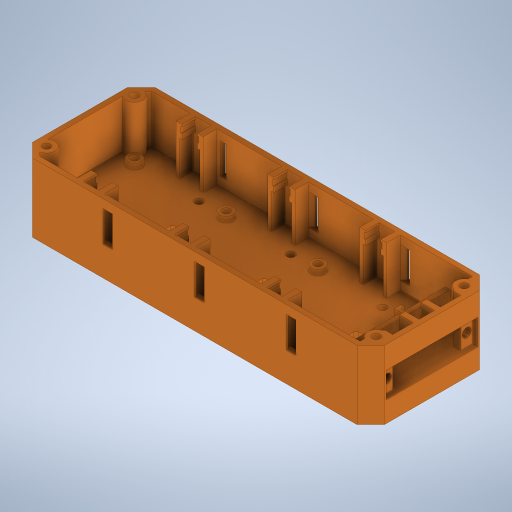
# Autodesk Inventor part: Sujecion
Saved by Autodesk Inventor 2024.2 (Build 282272000, 272)
## iProperties
Created: 2024-08-10
Part Number: Sujecion
Material: Generic
Document SubType Name: Modeling
Designer: Admin
Density: 1 g/cm^3
Appearance: Metal 1600F Hot
Author: Admin
Autodesk Inventor part; units mm, degrees
ref_plane "YZ Plane" through (0, 0, 0) normal (1, 0, 0) x (0, 1, 0)
ref_plane "XZ Plane" through (0, 0, 0) normal (0, 1, 0) x (-1, 0, 0)
sketch "Sketch1" plane through (0, 0, 0) normal (0, 1, 0) x (-1, 0, 0)
  line L0 (0, 0) -> (64, 0)
  line L1 (64, 0) -> (64, -72)
  line L2 (64, -72) -> (0, -72)
  line L3 (0, -72) -> (0, 0) construction
  line L4 (0, 0) -> (64, -72) construction
  line L5 (51, -17) -> (13, -17)
  line L6 (13, -17) -> (13, -55)
  line L7 (13, -55) -> (51, -55)
  line L8 (51, -55) -> (51, -17)
  line L9 (51, -17) -> (13, -55) construction
  line L10 (13, -17) -> (51, -55) construction
  circle A0 centre (51, -55) radius 1.6
  circle A1 centre (51, -17) radius 1.6
  circle A2 centre (13, -17) radius 1.6
  line L11 (10, -58) -> (54, -58) construction
  line L12 (54, -58) -> (54, -14) construction
  line L13 (54, -14) -> (10, -14) construction
  line L14 (10, -14) -> (10, -58) construction
  line L15 (10, -58) -> (54, -14) construction
  line L16 (54, -58) -> (10, -14) construction
  circle A3 centre (13, -55) radius 2.275
  circle A4 centre (-41, -55) radius 2.275
  line L17 (-41, -55) -> (-3, -55)
  circle A5 centre (-3, -55) radius 1.6
  line L18 (-44, -58) -> (0, -58) construction
  line L19 (-41, -17) -> (-41, -55)
  circle A6 centre (-41, -17) radius 1.6
  line L20 (-44, -14) -> (-44, -58) construction
  line L21 (10, -72) -> (-54, -72)
  line L22 (-3, -17) -> (-41, -55) construction
  line L23 (-3, -17) -> (-41, -17)
  line L24 (-3, -55) -> (-3, -17)
  line L25 (0, -58) -> (0, -14) construction
  line L26 (-44, -58) -> (0, -14) construction
  line L27 (0, -58) -> (-44, -14) construction
  line L28 (-54, -72) -> (-54, 0) construction
  line L29 (-54, 0) -> (10, -72) construction
  line L30 (-54, 0) -> (10, 0)
  line L31 (-41, -17) -> (-3, -55) construction
  circle A7 centre (-3, -17) radius 1.6
  line L32 (0, -14) -> (-44, -14) construction
  circle A8 centre (-95, -55) radius 2.275
  line L33 (-95, -55) -> (-57, -55)
  circle A9 centre (-57, -55) radius 1.6
  line L34 (-98, -58) -> (-54, -58) construction
  line L35 (-95, -17) -> (-95, -55)
  circle A10 centre (-95, -17) radius 1.6
  line L36 (-98, -14) -> (-98, -58) construction
  line L37 (-44, -72) -> (-108, -72)
  line L38 (-57, -17) -> (-95, -55) construction
  line L39 (-57, -17) -> (-95, -17)
  line L40 (-57, -55) -> (-57, -17)
  line L41 (-54, -58) -> (-54, -14) construction
  line L42 (-98, -58) -> (-54, -14) construction
  line L43 (-54, -58) -> (-98, -14) construction
  line L44 (-108, -72) -> (-108, 0) construction
  line L45 (-108, 0) -> (-44, -72) construction
  line L46 (-108, 0) -> (-44, 0)
  line L47 (-95, -17) -> (-57, -55) construction
  circle A11 centre (-57, -17) radius 1.6
  line L48 (-54, -14) -> (-98, -14) construction
  line L49 (-108, 0) -> (-143, 0)
  line L50 (-143, 0) -> (-143, -72)
  line L51 (-143, -72) -> (-108, -72)
  line L52 (-108, -72) -> (-108, 0) construction
  point P0 (32, -36)
  point P1 (-22, -36)
  point P2 (-76, -36)
  dimension "d0" = 64
  dimension "d1" = 72
  dimension "d2" = 38
  dimension "d3" = 38
  dimension "d6" = 3.2
  dimension "d9" = 180
  dimension "d11" = 44
  dimension "d12" = 44
  dimension "d13" = 4.55
  dimension "d21" = 54
  dimension "d26" = 35
  constraints: 106 end point, 12 centre point, 8 parallel, 6 coincident, 5 horizontal, 5 midpoint, 4 perpendicular, 1 collinear, 78 other
  measures "d0" distance of L0.start L0.end
  measures "d1" distance of L0.end L1.end
  measures "d2" distance of L7.end L5.start
  measures "d3" distance of L6.end L7.end
  measures "d6" diameter of A0
  measures "d11" distance of L13.end L12.end
  measures "d12" distance of L12.end L11.end
  measures "d13" diameter of A3
  measures "d21" distance of A3.centre A4.centre
  measures "d26" distance of L51.end L50.end
extrude "Base" add sketch "Sketch1" along normal blind 3.2 contours L0 L1 L2 L21 L37 L51 L50 L49 L46 L30 | L5 A1 L8 A0 L7 A3 L6 A2 | A4 L19 A6 L23 A7 L24 A5 L17 | A8 L35 A10 L39 A11 L40 A9 L33
sketch "Sketch2" plane through (0, 3.2, 0) normal (0, 1, 0) x (1, 0, 0)
  circle A0 centre (-13, 17) radius 1.6 projected
  line L0 (-13, 17) -> (-51, 55) construction
  circle A1 centre (-51, 55) radius 2.25
  circle A2 centre (-51, 55) radius 4
  line L1 (-32, 36) -> (-39.676, 28.324) construction
  circle A3 centre (-51, 17) radius 4
  circle A4 centre (-51, 17) radius 2.25
  circle A5 centre (-13, 17) radius 4
  circle A6 centre (-13, 17) radius 2.25
  line L2 (-64, 0) -> (143, 0) projected
  line L3 (-64, 0) -> (-54, 0)
  circle A7 centre (3, 17) radius 4
  circle A8 centre (3, 17) radius 2.25
  circle A9 centre (41, 17) radius 4
  circle A10 centre (41, 17) radius 2.25
  circle A11 centre (3, 55) radius 4
  circle A12 centre (3, 55) radius 2.25
  circle A13 centre (57, 17) radius 4
  circle A14 centre (57, 17) radius 2.25
  circle A15 centre (95, 17) radius 4
  circle A16 centre (95, 17) radius 2.25
  circle A17 centre (57, 55) radius 4
  circle A18 centre (57, 55) radius 2.25
  point P0 (0, 0)
  dimension "d29" = 4.5
  dimension "d30" = 8
  dimension "d33" = 180
  dimension "d38" = 54
  constraints: 18 centre point, 10 coincident, 6 end point, 1 horizontal, 1 midpoint, 1 point on line, 33 other
  measures "d29" diameter of A1
  measures "d30" diameter of A2
  measures "d38" distance of A3.centre A7.centre
extrude "EspacioInsertos" add sketch "Sketch2" along normal blind 3.2 contours A2 | A3 | A5 | A7 | A9 | A11 | A13 | A15 | A17
sketch "Sketch3" plane through (0, 3.2, 0) normal (0, 1, 0) x (1, 0, 0)
  circle A0 centre (-13, 17) radius 2.25 construction
  circle A1 centre (-51, 55) radius 2.25 construction
  line L0 (-13, 17) -> (-51, 55) construction
  line L1 (-54, 14) -> (-10, 14) construction
  line L2 (-10, 14) -> (-10, 58) construction
  line L3 (-10, 58) -> (-54, 58) construction
  line L4 (-54, 58) -> (-54, 14) construction
  line L5 (-54, 14) -> (-10, 58) construction
  line L6 (-10, 14) -> (-54, 58) construction
  line L7 (-9, 20.1) -> (-2.5, 20.1)
  line L8 (-2.5, 20.1) -> (-2.5, 35.6)
  line L9 (-2.5, 35.6) -> (-9, 35.6)
  line L10 (-9, 35.6) -> (-9, 20.1)
  line L11 (-9, 20.1) -> (-2.5, 35.6) construction
  line L12 (-2.5, 20.1) -> (-9, 35.6) construction
  line L13 (-64, 0) -> (143, 0) projected
  line L14 (-9, 21.6) -> (-7.5, 20.1)
  line L15 (-5.75, 27.85) -> (-7.0439, 27.85) construction
  line L16 (-5.75, 27.85) -> (-5.75, 26.4341) construction
  line L17 (-9, 34.1) -> (-7.5, 35.6)
  line L18 (-2.5, 21.6) -> (-4, 20.1)
  line L19 (-2.5, 34.1) -> (-4, 35.6)
  line L20 (45, 21.6) -> (46.5, 20.1)
  line L21 (45, 35.6) -> (45, 20.1)
  line L22 (45, 20.1) -> (51.5, 20.1)
  line L23 (51.5, 21.6) -> (50, 20.1)
  line L24 (51.5, 20.1) -> (51.5, 35.6)
  line L25 (51.5, 34.1) -> (50, 35.6)
  line L26 (51.5, 35.6) -> (45, 35.6)
  line L27 (45, 34.1) -> (46.5, 35.6)
  line L28 (0, 58) -> (0, 14) construction
  line L29 (0, 14) -> (44, 14) construction
  line L30 (44, 58) -> (0, 58) construction
  line L31 (44, 14) -> (44, 58) construction
  line L32 (99, 21.6) -> (100.5, 20.1)
  line L33 (99, 35.6) -> (99, 20.1)
  line L34 (99, 20.1) -> (105.5, 20.1)
  line L35 (105.5, 21.6) -> (104, 20.1)
  line L36 (105.5, 20.1) -> (105.5, 35.6)
  line L37 (105.5, 34.1) -> (104, 35.6)
  line L38 (105.5, 35.6) -> (99, 35.6)
  line L39 (99, 34.1) -> (100.5, 35.6)
  line L40 (54, 58) -> (54, 14) construction
  line L41 (54, 14) -> (98, 14) construction
  line L42 (98, 58) -> (54, 58) construction
  line L43 (98, 14) -> (98, 58) construction
  point P0 (0, 0)
  point P1 (-32, 36)
  dimension "d45" = 44
  dimension "d46" = 44
  dimension "d47" = 15.5
  dimension "d48" = 6.5
  dimension "d49" = 20.1
  dimension "d50" = 1
  dimension "d51" = 135
  dimension "d52" = 1.5
  dimension "d55" = 54
  constraints: 86 end point, 6 point on line, 6 symmetric about line, 5 midpoint, 4 parallel, 3 horizontal, 3 perpendicular, 1 vertical, 56 other
  measures "d45" distance of L3.end L2.end
  measures "d46" distance of L2.end L1.end
  measures "d47" distance of L9.end L7.start
  measures "d48" distance of L8.end L9.end
  measures "d49" distance between parallel lines of L13 L7
  measures "d50" distance between parallel lines of L10 L2
  measures "d51" angle of L14 L10
  measures "d52" horizontal distance of L14.start L14.end
  measures "d55" distance of L14.start L20.start
extrude "EntradaCables" cut sketch "Sketch3" against normal blind 3.2 contours L14 L10 L17 L9 L19 L8 L18 L7 | L21 L27 L26 L25 L24 L23 L22 L20 | L33 L39 L38 L37 L36 L35 L34 L32
sketch "Sketch4" plane through (0, 3.2, 0) normal (0, 1, 0) x (1, 0, 0)
  line L0 (-64, 72) -> (-64, 0) projected
  line L1 (143, 0) -> (143, 72) projected
  line L2 (-64, 72) -> (143, 72)
  line L3 (143, 72) -> (143, 0)
  line L4 (143, 0) -> (-64, 0)
  line L5 (-64, 0) -> (-64, 72)
  line L6 (143, 72) -> (-64, 72) projected
  line L7 (39.5, 72) -> (39.5, 36) construction
  line L8 (140, 69) -> (-61, 69)
  line L9 (-61, 69) -> (-61, 3)
  line L10 (-61, 3) -> (140, 3)
  line L11 (140, 3) -> (140, 69)
  line L12 (140, 69) -> (-61, 3) construction
  line L13 (-61, 69) -> (140, 3) construction
  point P0 (0, 0)
  dimension "d62" = 3
  dimension "d63" = 3
  dimension "d64" = 3
  constraints: 22 end point, 4 parallel, 3 midpoint, 2 horizontal, 2 perpendicular, 1 vertical
  measures "d62" distance between parallel lines of L9 L0
  measures "d63" distance between parallel lines of L4 L10
  measures "d64" distance between parallel lines of L2 L8
extrude "EliminacionExceso" add sketch "Sketch4" along normal blind 30
sketch "Sketch5" plane through (0, 3.2, 0) normal (0, 1, 0) x (1, 0, 0)
  circle A0 centre (-13, 17) radius 1.6 projected
  circle A1 centre (-51, 55) radius 4 projected
  line L0 (-13, 17) -> (-51, 55) construction
  line L1 (-54, 14) -> (-10, 14)
  line L2 (-10, 14) -> (-10, 58)
  line L3 (-10, 58) -> (-54, 58)
  line L4 (-54, 58) -> (-54, 14)
  line L5 (-54, 14) -> (-10, 58) construction
  line L6 (-10, 14) -> (-54, 58) construction
  line L7 (-61, 3) -> (140, 3) projected
  line L8 (-32.5, 3) -> (-16.5, 3)
  line L9 (-16.5, 3) -> (-16.5, 11)
  line L10 (-16.5, 11) -> (-32.5, 11)
  line L11 (-32.5, 11) -> (-32.5, 3)
  line L12 (37.5, 3) -> (37.5, 11)
  line L13 (37.5, 11) -> (21.5, 11)
  line L14 (21.5, 11) -> (21.5, 3)
  line L15 (21.5, 3) -> (37.5, 3)
  line L16 (91.5, 3) -> (91.5, 11)
  line L17 (91.5, 11) -> (75.5, 11)
  line L18 (75.5, 11) -> (75.5, 3)
  line L19 (75.5, 3) -> (91.5, 3)
  line L20 (143, 0) -> (143, 72) projected
  line L21 (143, 36) -> (123, 36) construction
  line L22 (-61, 69) -> (140, 69)
  line L23 (-32.5, 69) -> (-16.5, 69)
  line L24 (-16.5, 69) -> (-16.5, 61)
  line L25 (-16.5, 61) -> (-32.5, 61)
  line L26 (-32.5, 61) -> (-32.5, 69)
  line L27 (37.5, 69) -> (37.5, 61)
  line L28 (37.5, 61) -> (21.5, 61)
  line L29 (21.5, 61) -> (21.5, 69)
  line L30 (21.5, 69) -> (37.5, 69)
  line L31 (91.5, 69) -> (91.5, 61)
  line L32 (91.5, 61) -> (75.5, 61)
  line L33 (75.5, 61) -> (75.5, 69)
  line L34 (75.5, 69) -> (91.5, 69)
  point P0 (0, 0)
  point P1 (-32, 36)
  point P2 (91.5, 69)
  point P3 (75.5, 69)
  point P4 (37.5, 69)
  point P5 (21.5, 69)
  point P6 (-16.5, 69)
  dimension "d67" = 44
  dimension "d68" = 44
  dimension "d69" = 21.5
  dimension "d70" = 8
  dimension "d71" = 16
  dimension "d74" = 54
  constraints: 66 end point, 14 symmetric about line, 4 horizontal, 4 midpoint, 4 parallel, 2 perpendicular, 2 point on line, 16 other
  measures "d67" distance of L3.end L2.end
  measures "d68" distance of L2.end L1.end
  measures "d69" distance between parallel lines of L11 L4
  measures "d70" distance of L10.end L8.start
  measures "d71" distance of L9.end L10.end
  measures "d74" distance of L8.start L14.end
extrude "EspacioConectores" add sketch "Sketch5" along normal blind 30 contours L11 L10 L9 L7 | L14 L13 L12 L7 | L18 L17 L16 L7 | L22 L24 L25 L26 | L22 L27 L28 L29 | L22 L31 L32 L33
sketch "Sketch6" plane through (-16.5, 3.2, -11) normal (0, 0, -1) x (-1, 0, 0)
  line L0 (16, 0) -> (16, 30) projected
  line L1 (0, 0) -> (0, 30) projected
  line L2 (8, 30) -> (8, 27)
  line L3 (8, 30) -> (12.5, 30)
  line L4 (12.5, 30) -> (12.5, 27)
  line L5 (12.5, 27) -> (8, 27)
  line L6 (8, 27) -> (8, 30)
  line L7 (8, 27) -> (13.2, 27)
  line L8 (13.2, 27) -> (13.2, 23.5)
  line L9 (13.2, 23.5) -> (8, 23.5)
  line L10 (8, 23.5) -> (8, 27)
  line L11 (8, 23.5) -> (12.5, 23.5)
  line L12 (12.5, 23.5) -> (12.5, 20.5)
  line L13 (12.5, 20.5) -> (8, 20.5)
  line L14 (8, 20.5) -> (8, 23.5)
  line L15 (16, 0) -> (0, 0) projected
  line L16 (8, 20.5) -> (14, 20.5)
  line L17 (14, 20.5) -> (14, 0)
  line L18 (14, 0) -> (8, 0)
  line L19 (8, 0) -> (8, 20.5)
  line L20 (0, 0) -> (0, 30)
  line L21 (8, 30) -> (3.5, 30)
  line L22 (3.5, 30) -> (3.5, 27)
  line L23 (3.5, 27) -> (8, 27)
  line L24 (8, 27) -> (2.8, 27)
  line L25 (2.8, 27) -> (2.8, 23.5)
  line L26 (2.8, 23.5) -> (8, 23.5)
  line L27 (8, 23.5) -> (3.5, 23.5)
  line L28 (3.5, 23.5) -> (3.5, 20.5)
  line L29 (3.5, 20.5) -> (8, 20.5)
  line L30 (0, 0) -> (16, 0)
  line L31 (8, 20.5) -> (2, 20.5)
  line L32 (2, 20.5) -> (2, 0)
  line L33 (2, 0) -> (8, 0)
  point P0 (-16.5, -3.2)
  point P1 (2, 0)
  point P2 (12.5, 23.5)
  point P3 (3.5, 23.5)
  dimension "d84" = 4.5
  dimension "d85" = 5.2
  dimension "d86" = 3.5
  dimension "d88" = 3
  dimension "d89" = 3
  dimension "d90" = 6
  constraints: 62 end point, 10 symmetric about line, 8 parallel, 4 horizontal, 4 perpendicular, 2 point on line, 1 vertical
  measures "d84" distance of L4.end L5.end
  measures "d85" distance of L8.end L9.end
  measures "d86" distance of L7.end L8.end
  measures "d88" distance between parallel lines of L7 L3
  measures "d89" distance of L11.end L12.end
  measures "d90" distance of L17.end L18.end
extrude "EntradaConectores" cut sketch "Sketch6" against normal blind 8
pattern_linear "PatronConectoresI" count 3 spacing 54 along (1, 0, 0) of "EntradaConectores"
ref_plane "PlanoDivisor" through (0, 0, -36) normal (0, 0, 1) x (1, 0, 0)
mirror "PatronConectoresII" about plane through (0, 0, -36) normal (0, 0, 1) of "EntradaConectores", "PatronConectoresI"
sketch "Sketch7" plane through (0, 33.2, 0) normal (0, 1, 0) x (1, 0, 0)
  line L0 (-64, 0) -> (143, 0) projected
  line L1 (143, 0) -> (-64, 0)
  line L2 (-64, 0) -> (-64, 72)
  line L3 (-64, 72) -> (143, 72)
  line L4 (143, 72) -> (143, 0)
  point P0 (0, 0)
  constraints: 8 end point, 2 parallel, 1 horizontal, 1 perpendicular
extrude "DetalleSuperficialI" cut sketch "Sketch7" against normal blind 1.8
sketch "Sketch8" plane through (0, 3.2, 0) normal (0, 1, 0) x (1, 0, 0)
  line L0 (-64, 0) -> (-64, 72) projected
  line L1 (-64, 8) -> (-56, 0)
  line L2 (143, 0) -> (-64, 0) projected
  line L3 (-64, 8) -> (-64, 0)
  line L4 (-56, 0) -> (-64, 0)
  line L5 (-64, 36) -> (-49, 36) construction
  line L6 (-64, 12.2426) -> (-51.7574, 0)
  line L7 (-64, 72) -> (-64, 0)
  line L8 (-64, 64) -> (-56, 72)
  line L9 (143, 72) -> (-64, 72)
  line L10 (-64, 64) -> (-64, 72)
  line L11 (-56, 72) -> (-64, 72)
  line L12 (-64, 59.7574) -> (-51.7574, 72)
  line L13 (39.5, 72) -> (39.5, 42) construction
  line L14 (143, 0) -> (143, 72)
  line L15 (143, 8) -> (135, 0)
  line L16 (-64, 0) -> (143, 0)
  line L17 (143, 8) -> (143, 0)
  line L18 (135, 0) -> (143, 0)
  line L19 (143, 36) -> (128, 36) construction
  line L20 (143, 12.2426) -> (130.7574, 0)
  line L21 (143, 72) -> (143, 0)
  line L22 (143, 64) -> (135, 72)
  line L23 (-64, 72) -> (143, 72)
  line L24 (143, 64) -> (143, 72)
  line L25 (135, 72) -> (143, 72)
  line L26 (143, 59.7574) -> (130.7574, 72)
  point P0 (0, 0)
  point P1 (130.7574, 0)
  dimension "d99" = 135
  dimension "d100" = 8
  dimension "d102" = 3
  constraints: 50 end point, 23 symmetric about line, 16 point on line, 2 collinear, 2 midpoint, 1 horizontal, 1 parallel, 1 vertical
  measures "d99" angle of L0 L1
  measures "d100" horizontal distance of L1.start L1.end
  measures "d102" distance between parallel lines of L6 L1
extrude "DetalleSuperficialII" cut sketch "Sketch8" along normal through all both and the other way through all contours L0 L1 L2 | L0 L9 L8 | L15 L14 L2 | L9 L14 L22
extrude "Extrusion9" add sketch "Sketch8" along normal blind 28.2 contours L0 L6 L2 L1 | L0 L8 L9 L12 | L20 L14 L15 L2 | L9 L22 L14 L26
sketch "Sketch14" plane through (0, 3.2, 0) normal (0, 1, 0) x (1, 0, 0)
  line L0 (135, 72) -> (-56, 72) projected
  line L1 (121, 72) -> (121, 0)
  line L2 (143, 64) -> (143, 8) projected
  line L3 (118, 72) -> (118, 0)
  line L4 (118, 72) -> (121, 72)
  line L5 (118, 0) -> (121, 0)
  point P0 (0, 0)
  dimension "d117" = 22
  dimension "d118" = 3
  constraints: 8 end point, 2 parallel, 1 horizontal, 1 point on line, 1 vertical
  measures "d117" distance between parallel lines of L2 L1
  measures "d118" distance between parallel lines of L1 L3
extrude "EspacioFusible" add sketch "Sketch14" along normal blind 15
sketch "Sketch21" plane through (143, 0, -8) normal (1, 0, 0) x (0, 0, -1)
  line L0 (0, 31.4) -> (56, 31.4) projected
  line L1 (28, 31.4) -> (28, 0) construction
  line L2 (56, 0) -> (0, 0) projected
  line L3 (28, 0) -> (28, 3.2)
  line L4 (28, 3.2) -> (8, 3.2)
  line L5 (8, 3.2) -> (8, 18.2)
  line L6 (8, 18.2) -> (28, 18.2)
  line L7 (28, 18.2) -> (28, 3.2)
  line L8 (28, 3.2) -> (48, 3.2)
  line L9 (48, 3.2) -> (48, 18.2)
  line L10 (48, 18.2) -> (28, 18.2)
  point P0 (-8, 0)
  dimension "d138" = 3.2
  dimension "d139" = 20
  dimension "d140" = 15
  constraints: 18 end point, 2 midpoint, 2 parallel, 2 symmetric about line, 1 horizontal, 1 perpendicular, 1 point on line
  measures "d138" distance of L1.end L3.end
  measures "d139" distance of L5.end L6.end
  measures "d140" distance of L4.end L5.end
extrude "AccesoFusible" cut sketch "Sketch21" against normal blind 3
sketch "Sketch23" plane through (143, 0, -8) normal (1, 0, 0) x (0, 0, -1)
  line L0 (8, 18.2) -> (8, 3.2) construction
  line L1 (48, 3.2) -> (48, 18.2) construction
  line L2 (8, 18.2) -> (48, 18.2) construction
  line L3 (48, 18.2) -> (48, 3.2) construction
  line L4 (48, 3.2) -> (8, 3.2) construction
  line L5 (8, 3.2) -> (8, 18.2) construction
  line L6 (48, 18.2) -> (8, 3.2) construction
  circle A0 centre (28, 10.7) radius 2.25
  point P0 (-8, 0)
  dimension "d143" = 4.5
  constraints: 10 end point, 2 parallel, 1 centre point, 1 horizontal, 1 midpoint, 1 perpendicular
  measures "d143" diameter of A0
extrude "BarrenoFusible" cut sketch "Sketch23" against normal blind 30
sketch "Sketch24" plane through (0, 31.4, 0) normal (0, 1, 0) x (1, 0, 0)
  line L0 (121, 3) -> (121, 69) projected
  line L1 (121, 36) -> (131, 36) construction
  line L2 (121, 3) -> (133.7574, 3) projected
  line L3 (140, 9.2426) -> (140, 16) projected
  line L4 (133.7574, 3) -> (140, 9.2426)
  line L5 (140, 9.2426) -> (140, 16)
  line L6 (140, 16) -> (133.7574, 16)
  line L7 (133.7574, 16) -> (133.7574, 3)
  line L8 (140, 62.7574) -> (140, 56)
  line L9 (133.7574, 69) -> (140, 62.7574)
  line L10 (140, 62.7574) -> (140, 56)
  line L11 (140, 56) -> (133.7574, 56)
  line L12 (133.7574, 56) -> (133.7574, 69)
  point P0 (0, 0)
  constraints: 20 end point, 4 symmetric about line, 2 perpendicular, 1 collinear, 1 horizontal, 1 midpoint
extrude "SeccionMagnetos" add sketch "Sketch24" against normal blind 28.2
sketch "Sketch25" plane through (143, 0, -8) normal (1, 0, 0) x (0, 0, -1)
  line L0 (61, 18.2) -> (-5, 18.2) projected
  line L1 (55, 3.2) -> (1, 3.2)
  line L2 (1, 3.2) -> (1, 18.2)
  line L3 (1, 18.2) -> (55, 18.2)
  line L4 (55, 18.2) -> (55, 3.2)
  circle A0 centre (28, 10.7) radius 2.25 projected
  line L5 (55, 3.2) -> (1, 18.2) construction
  line L6 (1, 3.2) -> (55, 18.2) construction
  point P0 (-8, 0)
  dimension "d149" = 54
  constraints: 12 end point, 2 midpoint, 2 parallel, 1 horizontal, 1 perpendicular, 1 point on line
  measures "d149" distance of L2.end L3.end
extrude "EspacioTapa" cut sketch "Sketch25" against normal blind 3
sketch "Sketch28" plane through (0, 31.4, 0) normal (0, 1, 0) x (1, 0, 0)
  line L0 (-64, 64) -> (-64, 8) projected
  line L1 (-64, 36) -> (-69, 36) construction
  line L2 (-61, 9.2426) -> (-54.7574, 3) projected
  line L3 (-57.8787, 6.1213) -> (-57.8787, 65.8787) construction
  circle A0 centre (-57.8787, 10.1213) radius 2.25
  line L4 (-54.7574, 3) -> (-61, 9.2426) projected
  circle A1 centre (-57.8787, 10.1213) radius 5
  circle A2 centre (-57.8787, 61.8787) radius 2.25
  circle A3 centre (-57.8787, 61.8787) radius 5
  line L5 (0, 0) -> (-25.1943, 0) construction
  line L6 (-56, 0) -> (135, 0) projected
  circle A4 centre (136.1213, 10.1213) radius 5
  circle A5 centre (136.1213, 10.1213) radius 2.25
  circle A6 centre (136.1213, 61.8787) radius 5
  circle A7 centre (136.1213, 61.8787) radius 2.25
  dimension "d159" = 4.5
  dimension "d160" = 4
  dimension "d161" = 10
  dimension "d164" = 194
  constraints: 8 centre point, 6 end point, 3 midpoint, 2 horizontal, 2 point on line, 1 symmetric about line, 1 vertical, 8 other
  measures "d159" diameter of A0
  measures "d160" distance of point (-57.879, 6.121) A0.centre
  measures "d161" diameter of A1
  measures "d164" distance of A0.centre A4.centre
extrude "BarrenosTapaI" add sketch "Sketch28" against normal blind 28.2 contours A1 | A3
extrude "BarrenosTapaII" add sketch "Sketch28" against normal blind 10 contours A4 | A6
extrude "Extrusion25" cut sketch "Sketch28" against normal blind 10 contours A5 | A7
sketch "Sketch31" plane through (0, 0, 0) normal (0, -1, 0) x (1, 0, 0)
  line L0 (-56, 0) -> (-64, -8) projected
  line L1 (-56, 0) -> (-64, -8)
  line L2 (-64, -64) -> (-64, -8) projected
  line L3 (-64, -8) -> (-64, -64)
  line L4 (135, -72) -> (-56, -72) projected
  line L5 (-64, -64) -> (-56, -72)
  line L6 (135, -72) -> (143, -64) projected
  line L7 (-56, -72) -> (135, -72)
  line L8 (135, -72) -> (143, -64)
  line L9 (143, -64) -> (143, -8)
  line L10 (143, -8) -> (135, 0)
  line L11 (135, 0) -> (-56, 0)
  line L12 (-54.7574, -3) -> (-61, -9.2426)
  line L13 (-61, -9.2426) -> (-61, -62.7574)
  line L14 (-61, -62.7574) -> (-54.7574, -69)
  line L15 (-54.7574, -69) -> (133.7574, -69)
  line L16 (133.7574, -69) -> (140, -62.7574)
  line L17 (140, -62.7574) -> (140, -9.2426)
  line L18 (140, -9.2426) -> (133.7574, -3)
  line L19 (133.7574, -3) -> (-54.7574, -3)
  point P0 (0, 0)
  dimension "d181" = 3
  constraints: 32 end point, 8 perpendicular, 5 equal length, 7 other
  measures "d181" distance between parallel lines of L11 L19
extrude "Extrusion27" add sketch "Sketch31" along normal blind 9
sketch "Sketch26" plane through (140, 0, -8) normal (1, 0, 0) x (0, 0, -1)
  line L0 (55, 18.2) -> (55, 3.2) projected
  line L1 (1, 3.2) -> (1, 18.2) projected
  line L2 (48, 18.2) -> (8, 18.2) projected
  line L3 (8, 18.2) -> (8, 3.2) projected
  line L4 (8, 18.2) -> (8, 3.2)
  line L5 (48, 18.2) -> (48, 3.2)
  line L6 (44.725, 3.2) -> (49.275, 3.2) projected
  line L7 (55, 10.7) -> (48, 10.7) construction
  line L8 (8, 10.7) -> (1, 10.7) construction
  circle A0 centre (4.5, 10.7) radius 2.6
  line L9 (28, 18.2) -> (28, 15.2) construction
  circle A1 centre (51.5, 10.7) radius 2.6
  point P0 (-8, 0)
  dimension "d152" = 5.2
  constraints: 10 end point, 6 midpoint, 2 centre point, 2 vertical, 1 collinear, 1 point on line, 1 symmetric about line, 1 other
  measures "d152" diameter of A0
extrude "EspacioMagnetos" cut sketch "Sketch26" against normal blind 3.2
chamfer "Chamfer1" distance 2 angle 45 2 edges at (133.7574, 17.3, -16) (133.7574, 17.3, -56)
sketch "Sketch36" plane through (91.5, 3.2, -3) normal (0, 0, -1) x (-1, 0, 0)
  line L0 (0, 0) -> (0, 28.2) projected
  line L1 (0, 28.2) -> (0, 23.2)
  line L2 (0, 23.2) -> (-2, 23.2)
  line L3 (-2, 23.2) -> (-5.5, 23.2)
  line L4 (-5.5, 23.2) -> (-5.5, 5.2)
  line L5 (-5.5, 5.2) -> (-2, 5.2)
  line L6 (-2, 5.2) -> (-2, 23.2)
  line L7 (52, 5.2) -> (52, 23.2)
  line L8 (52, 23.2) -> (48.5, 23.2)
  line L9 (48.5, 23.2) -> (48.5, 5.2)
  line L10 (48.5, 5.2) -> (52, 5.2)
  line L11 (106, 5.2) -> (106, 23.2)
  line L12 (106, 23.2) -> (102.5, 23.2)
  line L13 (102.5, 23.2) -> (102.5, 5.2)
  line L14 (102.5, 5.2) -> (106, 5.2)
  point P0 (91.5, -3.2)
  dimension "d189" = 5
  dimension "d190" = 2
  dimension "d191" = 3.5
  dimension "d192" = 18
  dimension "d195" = 54
  constraints: 28 end point, 3 horizontal, 2 parallel, 1 collinear, 1 perpendicular, 1 point on line, 15 other
  measures "d189" distance of L0.end L1.end
  measures "d190" distance of L1.end L2.end
  measures "d191" distance of L5.end L4.end
  measures "d192" distance of L3.end L4.end
  measures "d195" distance of L5.end L7.start
extrude "Extrusion29" cut sketch "Sketch36" along normal mid plane 200
chamfer "Chamfer2" distance 2 angle 45 11 edges at (-11, 17.4, 0) (43, 17.4, 0) (97, 17.4, 0) (97, 17.4, -72) (43, 17.4, -72) (-11, 17.4, -72) (39.5, 17.4, -69) (93.5, 17.4, -69) (-14.5, 17.4, -3) (39.5, 17.4, -3) (93.5, 17.4, -3)
sketch "Sketch38" plane through (140, 31.4, -56) normal (-1, 0, 0) x (0, 0, 1)
  line L0 (40, 0) -> (0, 0) projected
  line L1 (20, 0) -> (20, -13.1691) construction
  line L2 (20, 0) -> (24.5, 0)
  line L3 (24.5, 0) -> (24.5, -3)
  line L4 (24.5, -3) -> (20, -3)
  line L5 (20, -3) -> (20, 0)
  line L6 (20, -3) -> (25.2, -3)
  line L7 (25.2, -3) -> (25.2, -6.5)
  line L8 (25.2, -6.5) -> (20, -6.5)
  line L9 (20, -6.5) -> (20, -3)
  line L10 (20, -6.5) -> (24.5, -6.5)
  line L11 (24.5, -6.5) -> (24.5, -9.5)
  line L12 (24.5, -9.5) -> (20, -9.5)
  line L13 (20, -9.5) -> (20, -6.5)
  line L14 (20, -9.5) -> (28, -9.5)
  line L15 (28, -9.5) -> (28, -13.2)
  line L16 (28, -13.2) -> (20, -13.2)
  line L17 (20, -13.2) -> (20, -9.5)
  line L18 (53, -13.2) -> (-13, -13.2) projected
  line L19 (20, 0) -> (28, 0)
  line L20 (28, 0) -> (28, -13.2)
  line L21 (28, -13.2) -> (20, -13.2)
  line L22 (20, -13.2) -> (20, 0)
  line L23 (0, 0) -> (40, 0)
  line L24 (20, 0) -> (15.5, 0)
  line L25 (15.5, 0) -> (15.5, -3)
  line L26 (15.5, -3) -> (20, -3)
  line L27 (20, -3) -> (14.8, -3)
  line L28 (14.8, -3) -> (14.8, -6.5)
  line L29 (14.8, -6.5) -> (20, -6.5)
  line L30 (20, -6.5) -> (15.5, -6.5)
  line L31 (15.5, -6.5) -> (15.5, -9.5)
  line L32 (15.5, -9.5) -> (20, -9.5)
  line L33 (20, -9.5) -> (12, -9.5)
  line L34 (12, -9.5) -> (12, -13.2)
  line L35 (12, -13.2) -> (20, -13.2)
  line L36 (20, 0) -> (12, 0)
  line L37 (12, 0) -> (12, -13.2)
  line L38 (14, -9.5) -> (14, -13.2)
  line L39 (26, -9.5) -> (26, -13.2)
  point P0 (56, -31.4)
  point P1 (15.5, -3)
  point P2 (15.5, 0)
  point P3 (12, -13.2)
  point P4 (15.5, -6.5)
  point P5 (24.5, -6.5)
  point P6 (24.5, -3)
  point P7 (15.5, 0)
  point P8 (15.5, -9.5)
  point P9 (24.5, -9.5)
  point P10 (15.5, -9.5)
  point P11 (24.5, -3)
  point P12 (15.5, -3)
  point P13 (24.5, -9.5)
  point P14 (14, -13.2)
  dimension "d206" = 4.5
  dimension "d207" = 3
  dimension "d208" = 3.5
  dimension "d209" = 3
  dimension "d210" = 5.2
  dimension "d212" = 3.7
  dimension "d213" = 3.5
  dimension "d217" = 2
  dimension "d218" = 2
  constraints: 76 end point, 12 symmetric about line, 10 parallel, 7 perpendicular, 5 horizontal, 5 point on line, 1 midpoint, 1 vertical
  measures "d206" distance of L1.start L2.end
  measures "d207" distance of L2.end L3.end
  measures "d208" distance of L6.end L7.end
  measures "d209" distance of L10.end L11.end
  measures "d210" distance of L7.end L8.end
  measures "d212" distance of L14.end L15.end
  measures "d213" distance between parallel lines of L20 L3
  measures "d217" distance between parallel lines of L37 L38
  measures "d218" distance between parallel lines of L15 L39
extrude "Extrusion30" add sketch "Sketch38" along normal blind 8 contours L20 L14 L11 L8 L7 L6 L3 L0 | L25 L27 L28 L29 L31 L33 L37 L0
sketch "Sketch39" plane through (0, 18.2, 0) normal (0, 1, 0) x (1, 0, 0)
  line L0 (118, 69) -> (118, 3) projected
  line L1 (118, 42.8275) -> (114, 42.8275)
  line L2 (114, 42.8275) -> (114, 44.8275)
  line L3 (114, 44.8275) -> (118, 44.8275)
  line L4 (118, 44.8275) -> (118, 42.8275)
  line L5 (114, 42.8275) -> (116, 42.8275)
  line L6 (116, 42.8275) -> (116, 46.8275)
  line L7 (116, 46.8275) -> (114, 46.8275)
  line L8 (114, 46.8275) -> (114, 42.8275)
  point P0 (0, 0)
  point P1 (116, 44.8275)
  dimension "d225" = 4
  dimension "d226" = 2
  dimension "d227" = 2
  dimension "d228" = 4
  constraints: 16 end point, 4 parallel, 2 horizontal, 2 perpendicular, 1 point on line
  measures "d225" distance of L2.end L3.end
  measures "d226" distance of L1.end L2.end
  measures "d227" distance of L7.end L6.end
  measures "d228" distance of L6.end L5.end
extrude "Extrusion31" add sketch "Sketch39" against normal through all
sketch "Sketch40" plane through (0, 0, 0) normal (0, -1, 0) x (1, 0, 0)
  line L0 (143, -9) -> (143, -63) projected
  line L1 (143, -36) -> (-64, -36) construction
  line L2 (-64, -8) -> (-64, -64) projected
  line L3 (-48, -66) -> (127, -66)
  line L4 (127, -66) -> (127, -6)
  line L5 (127, -6) -> (-48, -6)
  line L6 (-48, -6) -> (-48, -66)
  line L7 (-48, -66) -> (127, -6) construction
  line L8 (127, -66) -> (-48, -6) construction
  circle A0 centre (127, -6) radius 2.6
  circle A1 centre (127, -6) radius 5
  circle A2 centre (127, -66) radius 5
  circle A3 centre (127, -66) radius 2.6
  circle A4 centre (-48, -6) radius 5
  circle A5 centre (-48, -6) radius 2.6
  circle A6 centre (-48, -66) radius 5
  circle A7 centre (-48, -66) radius 2.6
  point P0 (0, 0)
  point P1 (39.5, -36)
  dimension "d229" = 5.2
  dimension "d230" = 10
  dimension "d231" = 60
  dimension "d232" = 175
  dimension "d235" = 60
  dimension "d238" = 175
  constraints: 14 end point, 8 centre point, 5 coincident, 5 midpoint, 2 horizontal, 2 parallel, 1 perpendicular, 1 vertical, 12 other
  measures "d229" diameter of A0
  measures "d230" diameter of A1
  measures "d231" distance of L3.end L4.end
  measures "d232" distance of L3.start L3.end
  measures "d235" distance of A1.centre A2.centre
  measures "d238" distance of A1.centre A4.centre
extrude "Extrusion32" add sketch "Sketch40" along normal blind 9 contours A7 L6 A6 L3 | L3 A6 L6 A7 | A2 L4 A3 L3 | L3 A3 L4 A2 | A4 L5 A5 L6 | L6 A5 L5 A4 | A1 L5 A0 L4 | L4 A0 L5 A1
extrude "Extrusion33" add sketch "Sketch40" along normal blind 5.8 contours L6 A7 L3 | L3 A7 L6 | A3 L4 L3 | L3 L4 A3 | A5 L5 L6 | L6 L5 A5 | A0 L5 L4 | L4 L5 A0
body "Solid1"
